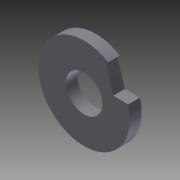
# Autodesk Inventor part: Gear Washer Spacer 2
Saved by Autodesk Inventor 2014 SP1 (Build 180222100, 222)
## iProperties
Created: 2012-03-30
Part Number: Gear Washer Spacer 2
Material: Steel
Document SubType Name: Modeling
Designer: Moses
Mass: 2.50667 g
Surface Area: 4.59642 cm^2
Volume: 0.319321 cm^3
Density: 7.85 g/cm^3
Appearance: Steel
Author: Moses
Autodesk Inventor part; units mm, degrees
ref_plane "YZ Plane" through (0, 0, 0) normal (1, 0, 0) x (0, 1, 0)
ref_plane "XZ Plane" through (0, 0, 0) normal (0, 1, 0) x (-1, 0, 0)
ref_plane "XY Plane" through (0, 0, 0) normal (0, 0, 1) x (1, 0, 0)
sketch "Sketch1" plane through (0, 0, 0) normal (0, 0, 1) x (1, 0, 0)
  circle A0 centre (0, 0) radius 7.9375
  circle A1 centre (0, 0) radius 3.175
  dimension "d0" = 15.875
  dimension "d1" = 6.35
  constraints: 2 centre point, 2 coincident
  measures "d0" diameter of A0
  measures "d1" diameter of A1
extrude "Extrusion1" add sketch "Sketch1" along normal blind 2.032
sketch "Sketch2" plane through (0, 0, 0) normal (0, 0, -1) x (-1, 0, 0)
  circle A0 centre (0, 0) radius 7.9375 construction
  arc A1 (-5.0493, 2.1833) -> (-17.7625, 1.0248) centre (-5.5945, -62.1721) ccw projected
  arc A2 (-3.7141, 6.4391) -> (-5.0493, 2.1833) centre (163.5858, -48.389) ccw projected
  arc A3 (-13.4868, 14.6525) -> (-3.7141, 6.4391) centre (32.6027, 59.5711) ccw projected
  arc A4 (-4.1702, 6.7537) -> (-7.6399, 2.1531) centre (0, 0) ccw
  constraints: 4 point on circle, 1 centre point, 1 coincident, 1 concentric
extrude "Extrusion2" cut sketch "Sketch2" against normal blind 25.4
body "Solid1"
